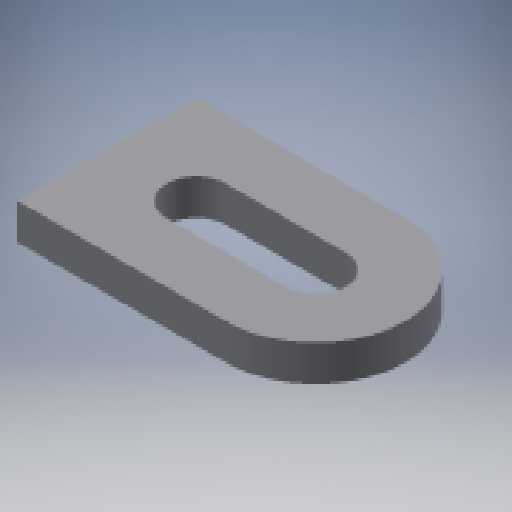
# Autodesk Inventor part: 24_0497_0019
Saved by Autodesk Inventor 2024.3 (Build 283343000, 343)
## iProperties
Created: 2024-06-17
Part Number: 24_0497_0019
Material: Allgemein
Document SubType Name: Modeling
Designer: Vogel
Density: 1 g/cm^3
Appearance: Vorgabe
Author: Vogel
Autodesk Inventor part; units mm, degrees
ref_plane "YZ Plane" through (0, 0, 0) normal (1, 0, 0) x (0, 1, 0)
ref_plane "XZ Plane" through (0, 0, 0) normal (0, 1, 0) x (-1, 0, 0)
ref_plane "XY Plane" through (0, 0, 0) normal (0, 0, 1) x (1, 0, 0)
sketch "Skizze1" plane through (0, 0, 0) normal (0, 0, 1) x (1, 0, 0)
  line L0 (-17.5, 0) -> (17.5, 0) projected
  line L1 (0, -10.5) -> (0, 10.5) projected
  line L2 (12.5, -7.5) -> (-12.5, -7.5)
  line L3 (-12.5, -7.5) -> (-12.5, 7.5)
  line L4 (-12.5, 7.5) -> (12.5, 7.5)
  line L5 (12.5, 7.5) -> (12.5, -7.5)
  line L6 (12.5, -7.5) -> (-12.5, 7.5) construction
  line L7 (-12.5, -7.5) -> (12.5, 7.5) construction
  point P0 (0, 0)
  dimension "d0" = 15
  dimension "d1" = 25
  constraints: 12 end point, 2 midpoint, 2 parallel, 1 horizontal, 1 perpendicular
  measures "d0" distance of L2.end L3.end
  measures "d1" distance of L3.end L4.end
extrude "Extrusion1" add sketch "Skizze1" along normal blind 2
fillet "Rundung1" radius 7.5 2 edges at (12.5, -7.5, 1) (12.5, 7.5, 1)
sketch "Skizze2" plane through (0, 0, 0) normal (0, 0, -1) x (-1, 0, 0)
  line L0 (17.5, 0) -> (-17.5, 0) projected
  line L1 (0, -10.5) -> (0, 10.5) projected
  line L2 (5, 0) -> (-5, 0) construction
  line L3 (5, 2.25) -> (-5, 2.25)
  line L4 (-5, -2.25) -> (5, -2.25)
  arc A0 (5, -2.25) -> (5, 2.25) centre (5, 0) ccw
  arc A1 (-5, 2.25) -> (-5, -2.25) centre (-5, 0) ccw
  point P0 (0, 0)
  dimension "d5" = 4.5
  dimension "d6" = 10
  constraints: 8 end point, 4 point on circle, 4 tangent, 2 centre point, 1 midpoint, 1 parallel, 1 point on line
  measures "d5" distance between parallel lines of L4 L3
  measures "d6" distance of L3.start L3.end
extrude "Extrusion2" cut sketch "Skizze2" against normal through all
